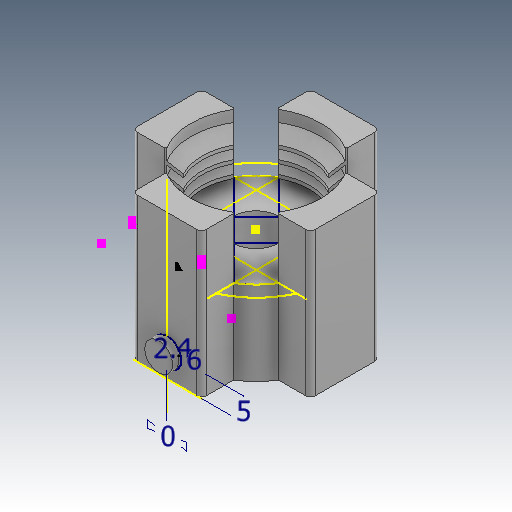
# Autodesk Inventor part: Slider V4-2 (spring with hole)
Saved by Autodesk Inventor 2021.3 (Build 253353000, 353)
## iProperties
Created: 2022-06-11
Part Number: Slider V4-2 (spring with hole)
Material: Generic
Document SubType Name: Modeling
Designer: david
Density: 1 g/cm^3
Appearance: Smooth - Medium Gray
Author: david
Autodesk Inventor part; units mm, degrees
ref_plane "YZ Plane" through (0, 0, 0) normal (1, 0, 0) x (0, 1, 0)
ref_plane "XZ Plane" through (0, 0, 0) normal (0, 1, 0) x (-1, 0, 0)
ref_plane "XY Plane" through (0, 0, 0) normal (0, 0, 1) x (1, 0, 0)
sketch "Sketch2" plane through (0, 0, 0) normal (0, 0, 1) x (1, 0, 0)
  line L0 (0, 0) -> (-11.557, 0) construction
  line L1 (0, -0.3685) -> (-13.97, -0.3685) construction
  line L2 (0, -1.2248) -> (-17.78, -1.2248) construction
  line L3 (-17.828, 0.4547) -> (-17.828, 16.3297)
  line L4 (-17.828, 16.3297) -> (-14.018, 16.3297)
  line L5 (-17.828, 0.4547) -> (-14.018, 0.4547)
  line L6 (-14.018, 0.4547) -> (-14.018, 5.6297)
  line L7 (-14.018, 5.6297) -> (-14.018, 7.6297)
  line L8 (-14.018, 7.6297) -> (-11.5904, 5.202)
  line L9 (-11.5904, 5.202) -> (-11.5904, 5.952)
  line L10 (-11.5904, 5.952) -> (-14.018, 8.3797)
  line L11 (-14.018, 8.3797) -> (-14.018, 10.3797)
  line L12 (-14.018, 10.3797) -> (-11.5904, 7.952)
  line L13 (-11.5904, 7.952) -> (-11.5904, 8.702)
  line L14 (-11.5904, 8.702) -> (-14.018, 11.1297)
  line L15 (-14.018, 11.1297) -> (-14.018, 13.1297)
  line L16 (-14.018, 13.1297) -> (-11.5904, 10.702)
  line L17 (-11.5904, 10.702) -> (-11.5904, 11.452)
  line L18 (-11.5904, 11.452) -> (-14.018, 13.8797)
  line L19 (-14.018, 16.3297) -> (-14.018, 13.8797)
  line L20 (0, -4.7358) -> (0, 19.8406) projected
  dimension "d2" = 11.557
  dimension "d3" = 13.97
  dimension "d4" = 0
  dimension "d5" = 17.78
  dimension "d6" = 0
  dimension "d7" = 15.875
  dimension "d8" = 3.81
  dimension "d9" = 5.175
  dimension "d10" = 2
  dimension "d11" = 45
  dimension "d12" = 2
  dimension "d13" = 0.75
  dimension "d14" = 45
  dimension "d15" = 0.75
  dimension "d21" = 2
  dimension "d23" = 0.75
  constraints: 40 end point, 8 vertical, 4 horizontal, 4 parallel, 2 point on line, 1 perpendicular
  measures "d2" distance of L0.start L0.end
  measures "d3" distance of L1.start L1.end
  measures "d4" horizontal distance of L0.start L1.start
  measures "d5" distance of L2.start L2.end
  measures "d6" horizontal distance of L0.start L2.start
  measures "d7" distance of L3.start L3.end
  measures "d8" distance of L3.start L5.end
  measures "d9" distance of L5.end L6.end
  measures "d10" distance of L6.end L7.end
  measures "d11" angle of L8 L7
  measures "d12" distance of L10.end L11.end
  measures "d13" distance of L8.end L9.end
  measures "d14" angle of L12 L11
  measures "d15" distance of L12.end L13.end
  measures "d21" distance of L14.end L15.end
  measures "d23" distance of L16.end L17.end
revolve "Revolution1" add sketch "Sketch2" angle 360 about axis through (0, -10, 0) along (0, 1, 0)
sketch "Sketch3" plane through (0, 0.4547, 0) normal (0, -1, 0) x (1, 0, 0)
  circle A0 centre (0, 0) radius 14.368
  circle A1 centre (0, 0) radius 17.828
  circle A2 centre (0, 0) radius 17.828 projected
  line L0 (7.45, -16.1968) -> (7.45, 16.1968)
  line L1 (0, 0) -> (0, 2.8388) construction
  line L2 (-7.45, -16.1968) -> (-7.45, 16.1968)
  line L3 (-7.45, -16.1968) -> (-7.45, -19.1968)
  line L4 (-7.45, -19.1968) -> (7.45, -19.1968)
  line L5 (7.45, -19.1968) -> (7.45, -16.1968)
  line L6 (0, 0) -> (2.0136, 0) construction
  line L7 (-7.45, 16.1968) -> (-7.45, 19.1968)
  line L8 (-7.45, 19.1968) -> (7.45, 19.1968)
  line L9 (7.45, 19.1968) -> (7.45, 16.1968)
  line L10 (19.1968, -7.45) -> (19.1968, 0)
  line L11 (19.1968, -7.45) -> (16.1968, -7.45)
  line L12 (16.1968, -7.45) -> (0, -7.45)
  line L13 (19.1968, 7.45) -> (19.1968, 0)
  line L14 (19.1968, 7.45) -> (16.1968, 7.45)
  line L15 (16.1968, 7.45) -> (0, 7.45)
  line L16 (-19.1968, -7.45) -> (-19.1968, 0)
  line L17 (-19.1968, -7.45) -> (-16.1968, -7.45)
  line L18 (-16.1968, -7.45) -> (0, -7.45)
  line L19 (-16.1968, 7.45) -> (0, 7.45)
  line L20 (-19.1968, 7.45) -> (-16.1968, 7.45)
  line L21 (-19.1968, 7.45) -> (-19.1968, 0)
  point P0 (-7.45, 12.2857)
  point P1 (-7.45, -12.2857)
  point P2 (7.45, -12.2857)
  point P3 (7.45, 12.2857)
  point P4 (-12.2857, 7.45)
  point P5 (-12.2857, -7.45)
  point P6 (12.2857, 7.45)
  point P7 (12.2857, -7.45)
  dimension "d27" = 7.45
  dimension "d44" = 3
  dimension "d65" = 7.45
  dimension "d66" = 0
  dimension "d67" = 3
  dimension "d73" = 28.736
  constraints: 44 end point, 12 symmetric about line, 4 vertical, 3 horizontal, 3 point on circle, 2 centre point, 2 coincident, 2 perpendicular
  measures "d27" distance from line of point (0, 0) L0
  measures "d44" distance of L4.end L0.start
  measures "d65" distance of L10.start L10.end
  measures "d66" vertical distance of point (0, 0) L10.end
  measures "d67" distance of L10.start L11.end
  measures "d73" diameter of A0
extrude "Extrusion1" add sketch "Sketch3" against normal blind 3 contours A0 L12 L0 L15 | L15 L0 A0 | A0 L0 L12 | L0 L15 L19 L2 A0 | L0 L12 L18 L2 L19 L15 | A0 L2 L18 L12 L0 | L2 L19 A0 | A0 L18 L2 | L19 L2 L18 A0
extrude "Extrusion2" cut sketch "Sketch3" against normal through all contours A0 L15 A1 L12 | A0 L0 A1 L15 | L12 A1 L0 A0 | A0 L19 A1 L2 | L2 A1 L18 A0 | A0 L18 A1 L19
extrude "Extrusion4" add sketch "Sketch3" against normal up to surface (15.875 mm away) contours A1 L7 L8 L9 | L5 L4 L3 A1
extrude "Extrusion9" add sketch "Sketch3" along normal blind 15.2 contours A0 L12 L0 L15 | L15 L0 A0 | A0 L0 L12 | L0 L15 L19 L2 A0 | A0 L2 A1 L0 | L0 L12 L18 L2 L19 L15 | L0 A1 L2 A0 | A0 L2 L18 L12 L0 | L2 L19 A0 | A1 L7 L8 L9 | A0 L18 L2 | L5 L4 L3 A1 | L19 L2 L18 A0
sketch "Sketch5" plane through (-7.45, 0.4547, 19.1968) normal (0, 0, 1) x (1, 0, 0)
  line L0 (-6.568, 9.925) -> (-6.568, 9.925) projected
  line L1 (-6.568, 10.675) -> (-6.568, 10.675) projected
  line L2 (21.468, 3) -> (21.468, 3) projected
  arc A0 (7.25, 3) -> (7.25, 3) centre (10.0691, 7.0273) ccw
  line L3 (14.9, -15.2) -> (0, -15.2) projected
  circle A1 centre (7.45, -10.2) radius 3
  line L4 (7.45, -21.415) -> (7.45, 22.09) projected
  arc A2 (4.6443, -9.138) -> (10.2691, -9.174) centre (7.4654, -7.8) ccw
  point P0 (14.9, 9.925)
  point P1 (0, 9.925)
  point P2 (14.9, 10.675)
  point P3 (0, 10.675)
  point P4 (-6.568, 3)
  dimension "d60" = 6
  dimension "d61" = 0
  dimension "d63" = 5
  dimension "d64" = 2.4
  constraints: 6 point on circle, 3 centre point, 6 other
  measures "d60" diameter of A1
  measures "d63" distance from line of L3 A1.centre
  measures "d64" vertical distance of A1.centre A2.centre
extrude "Extrusion6" add sketch "Sketch5" along normal blind 1.8 contours A1 L4 A2 | A2 L4 A1 | A1 A2 L4 | L4 A2 A1
extrude "Extrusion8" cut sketch "Sketch5" along normal blind 0.5 contours A1 L4 A2 | A1 A2 L4 picked at (7.9038, -11.6316) picked at (7.2108, -12.4117)
mirror "Mirror1" about plane through (0, 0, 0) normal (0, 0, 1) of "Extrusion6", "Extrusion8"
sketch "Sketch7" plane through (0, 3.4547, 0) normal (0, 1, 0) x (1, 0, 0)
  point P0 (0, 0)
  point P1 (0, 0)
  constraints: 1 coincident
hole "Hole1" at (0, 3.4547, 0) direction (0, -1, 0) diameter 5.3 end through all counterbore diameter 10 counterbore depth 12
extrude "Extrusion10" add sketch "Sketch3" along normal up to surface (15.2 mm away) contours A0 L15 A1 L12 | L14 L13 L10 L11 A1 | A0 L18 A1 L19 | A1 L17 L16 L21 L20
extrude "Extrusion11" add sketch "Sketch3" against normal up to surface (15.875 mm away) contours A0 L15 A1 L12 | L14 L13 L10 L11 A1 | A0 L18 A1 L19 | A1 L17 L16 L21 L20
fillet "Fillet1" radius 1 8 edges at (-19.1968, 0.7922, 7.45) (-19.1968, 0.7922, -7.45) (19.1968, 0.7922, 7.45) (19.1968, 0.7922, -7.45) (7.45, 0.7922, 19.1968) (-7.45, 0.7922, 19.1968) (-7.45, 0.7922, -19.1968) (7.45, 0.7922, -19.1968)
sketch "Sketch8" plane through (0, 3.4547, 0) normal (0, 1, 0) x (1, 0, 0)
  circle A0 centre (0, 0) radius 14.368 projected
  circle A1 centre (0, 0) radius 17.828 projected
  line L0 (7.45, 16.1968) -> (7.45, -16.1968) projected
  line L1 (16.1968, 7.45) -> (0, 7.45) projected
  line L2 (16.1968, -7.45) -> (0, -7.45) projected
  line L3 (-16.1968, -7.45) -> (0, -7.45) projected
  line L4 (-16.1968, 7.45) -> (0, 7.45) projected
  line L5 (-7.45, 16.1968) -> (-7.45, -16.1968) projected
  line L6 (-12.2857, -7.45) -> (-18.1968, -7.45) projected
  arc A2 (12.2857, 7.45) -> (7.45, 12.2857) centre (0, 0) ccw projected
  line L7 (-12.2857, -7.45) -> (7.45, 12.2857)
  line L8 (12.2857, 7.45) -> (18.1968, 7.45) projected
  line L9 (-7.45, -18.1968) -> (-7.45, -12.2857) projected
  line L10 (12.2857, 7.45) -> (-7.45, -12.2857)
  line L11 (18.1968, -7.45) -> (12.2857, -7.45) projected
  line L12 (-7.45, 12.2857) -> (-7.45, 18.1968) projected
  line L13 (12.2857, -7.45) -> (-7.45, 12.2857)
  arc A3 (-7.45, 12.2857) -> (-12.2857, 7.45) centre (0, 0) ccw projected
  line L14 (7.45, -12.2857) -> (7.45, -18.1968) projected
  line L15 (-12.2857, 7.45) -> (7.45, -12.2857)
  point P0 (-7.45, 12.2857)
  point P1 (-7.45, -7.45)
  point P2 (7.45, -7.45)
  point P3 (7.45, 7.45)
  point P4 (-7.45, 7.45)
  point P5 (0, -4.8357)
  point P6 (-4.8357, 0)
  point P7 (-12.2857, -7.45)
  point P8 (-7.45, -12.2857)
  point P9 (0, 4.8357)
  point P10 (-7.45, 12.2857)
  point P11 (-12.2857, 7.45)
  point P12 (12.2857, 7.45)
  point P13 (7.45, 12.2857)
  point P14 (4.8357, 0)
  point P15 (12.2857, -7.45)
  constraints: 8 end point, 2 other
extrude "Extrusion12" cut sketch "Sketch8" along normal through all contours L1 L0 A0 | A0 L0 L2 | L5 L4 A0 | A0 L3 L5
extrude "Extrusion13" cut sketch "Sketch8" along normal through all contours L10 L0 L1 | L2 L0 L13 | L0 L1 L7 | L0 L10 L13 L7 L1 | L15 L2 L0 | L2 L15 L10 L13 L0 | L13 L4 L5 | L5 L3 L10 | L4 L5 L15 | L4 L13 L7 L15 L5 | L10 L3 L5 L7 L15 | L7 L5 L3
equation "\"d15\" = d13"
equation "\"d23\" = d13"
body "Solid1"
